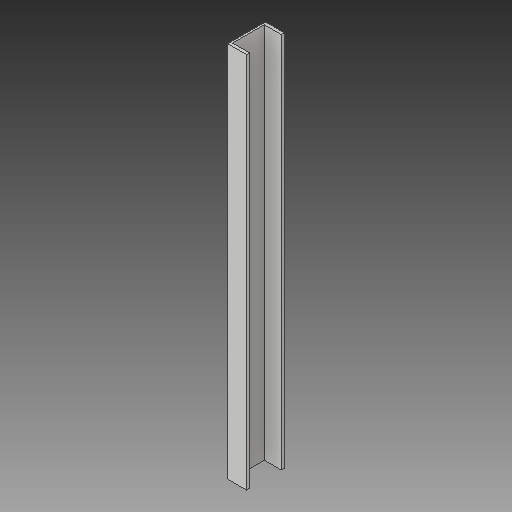
# Autodesk Inventor part: Channel1
Saved by Autodesk Inventor 2019 (Build 230136000, 136)
## iProperties
Created: 2019-05-26
Part Number: Channel1
Material: Generic
Document SubType Name: Modeling
Designer: dell
Density: 1 g/cm^3
Appearance: Default
Author: dell
Autodesk Inventor part; units mm, degrees
ref_plane "YZ Plane" through (0, 0, 0) normal (1, 0, 0) x (0, 1, 0)
ref_plane "XZ Plane" through (0, 0, 0) normal (0, 1, 0) x (-1, 0, 0)
ref_plane "XY Plane" through (0, 0, 0) normal (0, 0, 1) x (1, 0, 0)
sketch "Sketch1" plane through (0, 0, 0) normal (0, 1, 0) x (-1, 0, 0)
  line L0 (0, 0) -> (50, 0)
  line L1 (50, 0) -> (50, -100)
  line L2 (50, -100) -> (0, -100)
  line L3 (0, -100) -> (0, -92)
  line L4 (0, -92) -> (45, -92)
  line L5 (45, -92) -> (45, -8)
  line L6 (45, -8) -> (0, -8)
  line L7 (0, -8) -> (0, 0)
  dimension "d0" = 50
  dimension "d1" = 100
  dimension "d2" = 8
  dimension "d3" = 45
  dimension "d4" = 84
  constraints: 16 end point, 7 perpendicular, 1 horizontal, 1 point on line
  measures "d0" distance of L0.start L0.end
  measures "d1" distance of L0.end L1.end
  measures "d2" distance of L2.end L3.end
  measures "d3" distance of L3.end L4.end
  measures "d4" distance of L4.end L5.end
extrude "Extrusion1" add sketch "Sketch1" along normal blind 500
mirror "Mirror1" about plane through (-34.1154, 0, -50) normal (0, -1, 0) of "Extrusion1"
body "Solid1"
